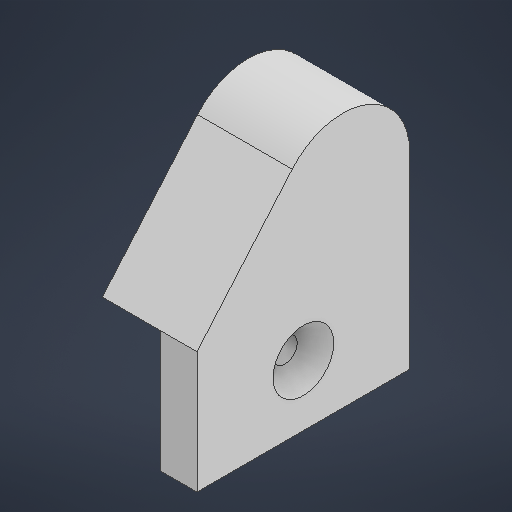
# Autodesk Inventor part: bearing_holder_v2_right
Saved by Autodesk Inventor 2026.2 (Build 302298000, 298)
## iProperties
Created: 2026-01-17
Part Number: bearing_holder_v2_right
Material: Generic
Document SubType Name: Modeling
Designer: User
Density: 1 g/cm^3
Appearance: Default
Author: User
Autodesk Inventor part; units mm, degrees
ref_plane "YZ Plane" through (0, 0, 0) normal (1, 0, 0) x (0, 1, 0)
ref_plane "XZ Plane" through (0, 0, 0) normal (0, 1, 0) x (-1, 0, 0)
ref_plane "XY Plane" through (0, 0, 0) normal (0, 0, 1) x (1, 0, 0)
sketch "Sketch1" plane through (0, 0, 0) normal (1, 0, 0) x (0, 1, 0)
  circle A0 centre (0, 0) radius 7
  line L0 (0, -11) -> (-31, -11)
  line L1 (-31, -11) -> (-31, 24)
  line L2 (-11, -11) -> (-11, 24)
  line L3 (-31, 24) -> (-11, 24)
  line L4 (0, -20.9958) -> (0, 31.4993) projected
  arc A1 (0, -11) -> (7.1808, 8.3329) centre (0, 0) ccw
  line L5 (-11, 24) -> (7.1808, 8.3329)
  dimension "d0" = 14
  dimension "d3" = 11
  dimension "d4" = 35
  dimension "d6" = 22
  dimension "d7" = 31
  constraints: 10 end point, 2 centre point, 2 horizontal, 2 point on circle, 2 point on line, 1 coincident, 1 parallel, 1 perpendicular, 1 tangent
  measures "d0" diameter of A0
  measures "d3" distance between parallel lines of L2 L4
  measures "d4" distance of L0.end L1.end
  measures "d6" diameter of A1
  measures "d7" distance from line of L1 point (0, 0)
extrude "Extrusion1" add sketch "Sketch1" along normal blind 9.5813 contours A0 L4 L5 A1 | A0 L4 L0 L2 L5
extrude "Extrusion2" add sketch "Sketch1" along normal blind 4.5813 contours A0 L4 | L4 A0
extrude "Extrusion3" add sketch "Sketch1" against normal blind 6
mirror "Mirror1" about plane through (9.5813, 0, 6.5) normal (1, 0, 0) of "Extrusion1", "Extrusion2", "Extrusion3"
sketch "Sketch2" plane through (0, -31, 24) normal (0, 0, 1) x (1, 0, 0)
  line L0 (-6, 31) -> (-6, 0) projected
  line L1 (-6, 0) -> (9.5813, 0)
  line L2 (9.5813, 0) -> (9.5813, 45.1625)
  line L3 (9.5813, 45.1625) -> (-6, 45.1625)
  line L4 (-6, 45.1625) -> (-6, 0)
  point P0 (0, 31)
  constraints: 8 end point, 2 parallel, 1 horizontal, 1 perpendicular
extrude "Extrusion4" cut sketch "Sketch2" against normal through all
sketch "Sketch3" plane through (25.1625, -31, -11) normal (1, 0, 0) x (0, 0, -1)
  circle A0 centre (-17.5, 10) radius 2
  line L0 (-35, 0) -> (-35, 20) projected
  line L1 (0, 0) -> (-35, 0) projected
  point P0 (-11, 31)
  point P1 (-35, 10)
  point P2 (-17.5, 0)
  dimension "d16" = 4
  dimension "d17" = 0
  dimension "d18" = 0
  constraints: 2 midpoint, 1 centre point
  measures "d16" diameter of A0
  measures "d17" vertical distance of point (-35, 10) A0.centre
  measures "d18" horizontal distance of point (-17.5, 0) A0.centre
extrude "Extrusion5" cut sketch "Sketch3" against normal blind 10
chamfer "Chamfer1" distance 3 angle 45 1 edges at (25.1625, -21, 8.5)
body "Solid1"
